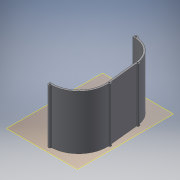
# Autodesk Inventor part: case bottom half
Saved by Autodesk Inventor 2017 (Build 210142000, 142)
## iProperties
Created: 2018-04-17
Part Number: case bottom half
Material: Generic
Document SubType Name: Modeling
Designer: RKL
Density: 1 g/cm^3
Appearance: Default
Author: RKL
Autodesk Inventor part; units mm, degrees
ref_plane "YZ Plane" through (0, 0, 0) normal (1, 0, 0) x (0, 1, 0)
ref_plane "XZ Plane" through (0, 0, 0) normal (0, 1, 0) x (-1, 0, 0)
ref_plane "XY Plane" through (0, 0, 0) normal (0, 0, 1) x (1, 0, 0)
ref_plane "Work Plane1" through (0, 0, 0) normal (0, 0, 1) x (1, 0, 0)
sketch "Sketch1" plane through (0, 0, 0) normal (0, 0, 1) x (1, 0, 0)
  circle A0 centre (-55.8916, -14.7421) radius 1.397 projected
  circle A1 centre (-83.8916, 18.2579) radius 1.397 projected
  circle A2 centre (-83.8916, -14.7421) radius 1.397 projected
  circle A3 centre (-55.8916, 18.2579) radius 1.397 projected
  circle A4 centre (2.1895, 105.4705) radius 1.905 projected
  circle A5 centre (-2.169, -104.4843) radius 1.905 projected
  circle A6 centre (60.6164, 51.7463) radius 1.905 projected
  circle A7 centre (-58.4167, 54.2173) radius 1.905 projected
  arc A8 (6.1836, 105.2542) -> (-1.8102, 105.4201) centre (2.1895, 105.4705) ccw projected
  arc A9 (-1.8102, 105.4201) -> (-57.7029, 58.1531) centre (0.9442, 45.4834) ccw construction
  arc A10 (-57.7029, 58.1531) -> (-58.999, 50.2599) centre (-58.4167, 54.2173) ccw projected
  line L0 (-58.999, 50.2599) -> (-63.1925, 21.7579) projected
  line L1 (-87.8916, 21.7579) -> (-63.1925, 21.7579) projected
  line L2 (-87.8916, -18.2421) -> (-87.8916, 21.7579) projected
  line L3 (-87.8916, -18.2421) -> (-73.1277, -26.766) projected
  arc A11 (-73.1277, -26.766) -> (-70.4395, -28.2823) centre (-69.9706, -24.3098) ccw projected
  arc A12 (-70.4395, -28.2823) -> (-6.1641, -104.2871) centre (-0.7162, -34.4994) ccw construction
  arc A13 (-6.1641, -104.2871) -> (1.8309, -104.453) centre (-2.169, -104.4843) ccw projected
  arc A14 (1.8309, -104.453) -> (69.2051, -31.1811) centre (-0.7162, -34.4994) ccw projected
  arc A15 (69.2051, -31.1811) -> (68.4839, -23.2145) centre (68.9014, -27.1927) ccw projected
  line L4 (68.4839, -23.2145) -> (61.034, 47.7681) projected
  arc A16 (61.034, 47.7681) -> (60.0665, 55.7083) centre (60.6164, 51.7463) ccw projected
  arc A17 (60.0665, 55.7083) -> (6.1836, 105.2542) centre (0.9442, 45.4834) ccw projected
  circle A18 centre (-69.9706, -24.3098) radius 1.905 projected
  circle A19 centre (68.9014, -27.1927) radius 1.905 projected
  circle A20 centre (0.9442, 45.4834) radius 17.5 projected
  circle A21 centre (-0.7162, -34.4994) radius 17.5 projected
  circle A22 centre (-66.7556, 10.6536) radius 4 projected
  circle A23 centre (-75.8916, -7.1378) radius 4 projected
  line L5 (-6.1641, -104.2871) -> (-1.8102, 105.4201) construction
  line L6 (-6.1641, -104.2871) -> (-6.0811, -100.2871)
  line L7 (-1.8102, 105.4201) -> (-1.8933, 101.4201)
  arc A24 (-6.0811, -100.2871) -> (64.9295, -27.6117) centre (-0.7162, -34.4994) ccw
  arc A25 (56.6471, 51.3278) -> (-1.8933, 101.4201) centre (0.9442, 45.4834) ccw
  line L8 (64.9295, -27.6117) -> (56.6471, 51.3278)
  point P0 (0, 0)
  dimension "d0" = 4
  dimension "d1" = 4
  constraints: 8 end point, 4 point on circle, 2 centre point, 2 coincident, 2 point on line, 2 tangent
  measures "d0" vertical distance of L5.end L7.end
  measures "d1" vertical distance of L5.start L6.end
extrude "Extrusion1" add sketch "Sketch1" along normal blind 135 contours A17 A16 L4 A15 A14 A13 L6 A24 L8 A25 L7 A8
body "Solid1"
